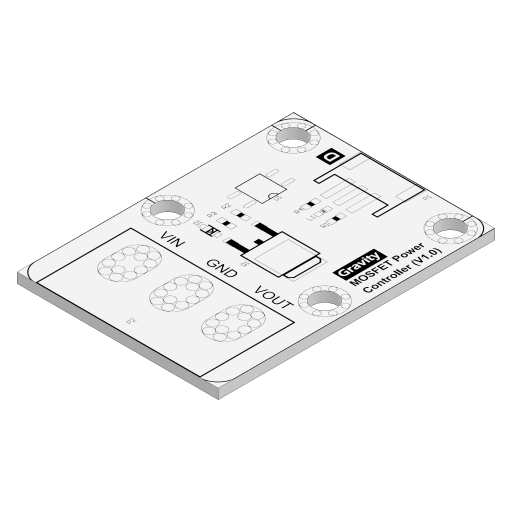
# Autodesk Inventor part: DFR-08104
Saved by Autodesk Inventor 2024.3 (Build 283343000, 343)
## iProperties
Created: 2025-06-26
Part Number: DFR-08104
Material: Generic
Document SubType Name: Modeling
Designer: MPA
Density: 1 g/cm^3
Appearance: Default
Author: MPA
Autodesk Inventor part; units mm, degrees
ref_plane "YZ Plane" through (0, 0, 0) normal (1, 0, 0) x (0, 1, 0)
ref_plane "XZ Plane" through (0, 0, 0) normal (0, 1, 0) x (-1, 0, 0)
ref_plane "XY Plane" through (0, 0, 0) normal (0, 0, 1) x (1, 0, 0)
sketch "Sketch1" plane through (0, 0, 0) normal (0, 1, 0) x (-1, 0, 0)
  line L0 (0, 0) -> (0, -44) construction
  line L1 (0, -44) -> (-31.9955, -44) construction
  line L2 (-31.9955, -44) -> (-31.9955, 0) construction
  line L3 (-31.9955, 0) -> (0, 0) construction
  dimension "d5" = 44
  dimension "d9" = 31.9955
  constraints: 1 coincident, 2 other
  measures "d5" distance of L0.start L0.end
  measures "d9" distance of L0.end L1.end
sketch "Sketch2" plane through (0, 0, 0) normal (0, 1, 0) x (-1, 0, 0)
  line L0 (0, 0) -> (0, -44) construction
  line L1 (0, -44) -> (-31.9955, -44) construction
  line L2 (-31.9955, -44) -> (-31.9955, 0) construction
  line L3 (-31.9955, 0) -> (0, 0) construction
  line L4 (0, 0) -> (-31.9955, 0)
  line L5 (-31.9955, 0) -> (-31.9955, -44)
  line L6 (-31.9955, -44) -> (0, -44)
  line L7 (0, -44) -> (0, 0)
  constraints: 8 end point, 2 parallel, 1 horizontal, 1 perpendicular
extrude "Extrusion1" add sketch "Sketch2" against normal blind 1.6
decal "Decal1"
sketch "Sketch4" plane through (0, 0, 0) normal (0, 1, 0) x (1, 0, 0)
  line L0 (3.4199, 20.4831) -> (28.4199, 20.4831)
  line L1 (28.4199, 20.4831) -> (28.4199, 40.4831)
  line L2 (28.4199, 40.4831) -> (3.4199, 40.4831)
  line L3 (3.4199, 40.4831) -> (3.4199, 20.4831)
  line L4 (3.4199, 20.4831) -> (28.4199, 40.4831) construction
  line L5 (28.4199, 20.4831) -> (3.4199, 40.4831) construction
  point P0 (0, 0)
  point P1 (15.9199, 30.4831)
  dimension "d14" = 25
  dimension "d15" = 20
  constraints: 12 end point, 4 coincident, 2 midpoint, 2 parallel, 1 horizontal, 1 perpendicular
  measures "d14" distance of L2.end L1.end
  measures "d15" distance of L1.end L0.end
hole "Hole1" at (3.4199, 0, -40.4831) at (3.4199, 0, -20.4831) at (28.4199, 0, -20.4831) at (28.4199, 0, -40.4831) direction (0, -1, 0) diameter 3.9 depth 3
body "Solid1"
